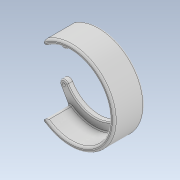
# Autodesk Inventor part: hip_back_motor_protector
Saved by Autodesk Inventor 2020 (Build 240168000, 168)
## iProperties
Created: 2021-01-28
Part Number: hip_back_motor_protector
Material: Generic
Document SubType Name: Modeling
Designer: DELL
Density: 1 g/cm^3
Appearance: Default
Author: DELL
Autodesk Inventor part; units mm, degrees
ref_plane "YZ Plane" through (0, 0, 0) normal (1, 0, 0) x (0, 1, 0)
ref_plane "XZ Plane" through (0, 0, 0) normal (0, 1, 0) x (-1, 0, 0)
ref_plane "XY Plane" through (0, 0, 0) normal (0, 0, 1) x (1, 0, 0)
sketch "Sketch1" plane through (0, 0, 0) normal (0, 0, 1) x (1, 0, 0)
  circle A0 centre (0, 0) radius 31.5
  circle A1 centre (0, 0) radius 40
  circle A2 centre (0, 0) radius 36 construction
  circle A3 centre (0, 0) radius 45
  line L0 (0, 0) -> (-38.9711, 22.5) construction
  line L1 (0, 0) -> (-38.9711, -22.5) construction
  line L2 (0, 0) -> (38.9711, 22.5) construction
  line L3 (0, 0) -> (38.9711, -22.5) construction
  line L4 (-45, 0) -> (45, 0) construction
  line L5 (0, 45) -> (0, -45) construction
  circle A4 centre (-31.1769, 18) radius 1.65
  circle A5 centre (-31.1769, -18) radius 1.65
  circle A6 centre (31.1769, -18) radius 1.65
  circle A7 centre (31.1769, 18) radius 1.65
  line L6 (-34.641, 20) -> (-24.3333, 37.8536)
  line L7 (-34.641, -20) -> (-24.3333, -37.8536)
  circle A8 centre (-30.9604, 17.875) radius 4.25
  circle A9 centre (-30.9604, -17.875) radius 4.25
  point P0 (-27.2798, 15.75)
  point P1 (-27.2798, -15.75)
  dimension "d1" = 90
  dimension "d0" = 80
  dimension "d2" = 63
  dimension "d3" = 72
  dimension "d4" = 30
  dimension "d5" = 30
  dimension "d6" = 3.3
  constraints: 16 end point, 9 centre point, 8 point on line, 6 point on circle, 6 tangent, 4 coincident, 4 midpoint, 3 equal radius, 1 horizontal, 1 vertical, 14 other
  measures "d0" diameter of A1
  measures "d2" diameter of A0
  measures "d3" diameter of A2
  measures "d4" angle of L4 L0
  measures "d5" angle of L4 L1
  measures "d6" diameter of A4
extrude "Extrusion1" add sketch "Sketch1" along normal blind 6 contours A0 A8 A1 A9 | A8 | A9 | L6 A3 L7 A1 picked at (33.8086, -10.8471) picked at (23.161, -34.4452)
extrude "Extrusion2" add sketch "Sketch1" along normal blind 25 from surface at 6 contours L6 A3 L7 A1 picked at (23.161, -34.4452)
fillet "Fillet1" radius 2 7 edges at (-34.641, 20, 18.5) (-34.641, -20, 18.5) (40, 0, 31) (45, 0, 31) (45, 0, 0) (-24.3333, 37.8536, 15.5) (-24.3333, -37.8536, 15.5)
fillet "Fillet2" radius 1 3 edges at (-25.3186, 33.0198, 6) (-25.3186, -33.0198, 6) (40, 0, 6)
fillet "Fillet3" radius 1 12 edges at (-30.7279, -26.7777, 6) (-26.2241, -34.5785, 6.3262) (-26.2241, 34.5785, 6.3262) (-30.7279, 26.7777, 6) (-30.6961, -26.8328, 0) (-25.1053, -36.5163, 0.4921) (-26.2215, -34.583, 0.0404) (-24.2813, -37.8219, 1.5354) (-26.2215, 34.583, 0.0404) (-25.1053, 36.5163, 0.4921) (-24.2813, 37.8219, 1.5354) (-30.6961, 26.8328, 0)
body "Solid1"
